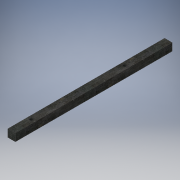
# Autodesk Inventor part: Base395
Saved by Autodesk Inventor 2019 (Build 230136000, 136)
## iProperties
Created: 2021-03-22
Part Number: Base395
Material: Steel
Document SubType Name: Modeling
Designer: User
Density: 7.85 g/cm^3
Appearance: Plate
Author: User
Autodesk Inventor part; units mm, degrees
ref_plane "YZ Plane" through (0, 0, 0) normal (1, 0, 0) x (0, 1, 0)
ref_plane "XZ Plane" through (0, 0, 0) normal (0, 1, 0) x (-1, 0, 0)
ref_plane "XY Plane" through (0, 0, 0) normal (0, 0, 1) x (1, 0, 0)
sketch "Sketch1" plane through (0, 0, 0) normal (0, 1, 0) x (-1, 0, 0)
  line L0 (0, 0) -> (19, 0)
  line L1 (19, 0) -> (19, -395)
  line L2 (19, -395) -> (0, -395)
  line L3 (0, -395) -> (0, 0)
  dimension "d0" = 19
  dimension "d1" = 395
  constraints: 8 end point, 2 parallel, 1 horizontal, 1 perpendicular
  measures "d0" distance between parallel lines of L1 L3
  measures "d1" distance between parallel lines of L2 L0
extrude "Extrusion1" add sketch "Sketch1" along normal mid plane 19
sketch "Sketch2" plane through (0, 9.5, 0) normal (0, 1, 0) x (1, 0, 0)
  circle A0 centre (-9.5, 50) radius 4
  circle A1 centre (-9.5, 285) radius 4
  line L0 (-19, 0) -> (0, 0) projected
  line L1 (-19, 395) -> (-19, 0) projected
  line L2 (0, 395) -> (-19, 395) projected
  dimension "d4" = 8
  dimension "d5" = 8
  dimension "d6" = 50
  dimension "d7" = 9.5
  dimension "d8" = 9.5
  dimension "d12" = 235
  constraints: 2 centre point
  measures "d4" diameter of A0
  measures "d5" diameter of A1
  measures "d6" distance from line of A0.centre L0
  measures "d7" distance from line of L1 A0.centre
  measures "d8" distance from line of L1 A1.centre
  measures "d12" distance of A1.centre A0.centre
extrude "Extrusion2" cut sketch "Sketch2" against normal blind 19
body "Solid1"
